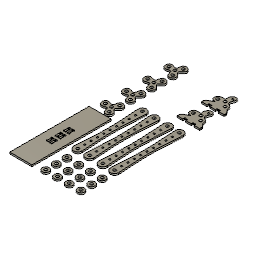
yufeng-lamp-thing (Autodesk Fusion 360 design; units mm, degrees)
part number: 2025-10-18-16-30-31-717
Autodesk Fusion 360 part; units mm, degrees
box "BoxPrimitive1" add length 1219.2 width 2438.4 height 11.7856 placed x (0, -1, 0) y (1, 0, 0) z (0, 0, 1) at (-34.3572, 8.0961, 0) makes body 1
move_body "Move1" bodies 1 to x (1, 0, 0) y (0, 1, 0) z (0, 0, 1) at (-89.6703, 115.0941, 0)
move_body "Move2" bodies 1 to x (1, 0, 0) y (0, 1, 0) z (0, 0, 1) at (127.2488, 1.4769, 0)
move_body "Move3" bodies 1 to x (1, 0, 0) y (0, 1, 0) z (0, 0, 1) at (-10.4658, -136.055, 0)
sketch "ELBOW" plane through (0, 0, 0) normal (0, 0, 1) x (1, 0, 0)
  line L0 (222.5472, -135.4361) -> (185.0472, -70.4842) construction
  line L1 (185.0472, -70.4842) -> (147.5472, -135.4361) construction
  line L2 (147.5472, -135.4361) -> (222.5472, -135.4361) construction
  circle A0 centre (185.0472, -70.4842) radius 25 construction
  circle A1 centre (147.5472, -135.4361) radius 25 construction
  circle A2 centre (222.5472, -135.4361) radius 25 construction
  line L3 (147.5472, -135.4361) -> (122.5472, -135.4361) construction
  line L4 (147.5472, -135.4361) -> (135.0472, -157.0867) construction
  line L5 (185.0472, -70.4842) -> (172.5472, -48.8336) construction
  line L6 (185.0472, -70.4842) -> (197.5472, -48.8336) construction
  line L7 (222.5472, -135.4361) -> (235.0472, -157.0867) construction
  line L8 (222.5472, -135.4361) -> (247.5472, -135.4361) construction
  line L9 (160.0472, -70.4842) -> (210.0472, -70.4842) construction
  line L10 (135.0472, -113.7855) -> (160.0472, -157.0867) construction
  line L11 (235.0472, -113.7855) -> (210.0472, -157.0867) construction
  line L12 (222.5472, -135.4361) -> (166.2972, -102.9601) construction
  line L13 (147.5472, -135.4361) -> (203.7972, -102.9601) construction
  line L14 (185.0472, -70.4842) -> (185.0472, -135.4361) construction
  spline S0 degree 5 poles (135.0472, -113.7855) (136.2523, -113.2432) (138.7814, -112.2557) (142.8843, -111.0513) (148.7127, -109.8794) (155.7527, -108.6478) (161.6818, -107.0834) (165.7867, -104.6636) (167.6575, -101.0152) (167.4018, -96.0557) (165.6038, -89.9888) (163.1024, -83.1934) (160.8198, -76.1444) (159.5754, -69.3217) (159.8917, -63.1196) (161.8468, -57.7723) (165.2277, -53.3996) (169.6524, -50.0384) (174.6931, -47.6782) (180.0245, -46.2985) (185.4687, -45.8896) (190.9043, -46.448) (196.2048, -47.9783) (201.1762, -50.4916) (205.4677, -54.0091) (208.6506, -58.5364) (210.3608, -64.026) (210.421, -70.343) (208.9713, -77.23) (206.5972, -84.2719) (204.1437, -90.9845) (202.5341, -96.9015) (202.5772, -101.6663) (204.8014, -105.1107) (209.2243, -107.369) (215.3774, -108.8454) (222.513, -110.0767) (229.759, -111.6244) (236.2898, -113.9581) (241.5029, -117.3331) (245.1562, -121.6999) (247.2527, -126.8142) (247.9512, -132.3267) (247.4748, -137.8722) (246.004, -143.1792) (243.6359, -148.0984) (240.4346, -152.5265) (236.459, -156.3518) (231.7968, -159.4005) (226.6048, -161.3583) (221.0926, -161.8511) (215.4834, -160.5874) (209.9826, -157.481) (204.7431, -152.782) (199.8317, -147.2051) (195.2451, -141.724) (190.9257, -137.3715) (186.7777, -135.0265) (182.6827, -135.2305) (178.5155, -137.9316) (174.1603, -142.5222) (169.5261, -148.0862) (164.5628, -153.5876) (159.2764, -158.0765) (153.7471, -160.9037) (148.1386, -161.8842) (142.6612, -161.1426) (137.5381, -158.9913) (132.9737, -155.806) (129.1131, -151.8787) (126.0369, -147.3683) (123.8027, -142.3818) (122.4778, -137.0263) (122.1686, -131.4643) (123.0691, -125.989) (125.3984, -120.9688) (128.5177, -117.5882) (131.5508, -115.5095) (133.8421, -114.3278) (135.0472, -113.7855) knots 0 0 0 0 0 0 0.01333333 0.02666667 0.04 0.05333333 0.06666667 0.08 0.09333333 0.10666667 0.12 0.13333333 0.14666667 0.16 0.17333333 0.18666667 0.2 0.21333333 0.22666667 0.24 0.25333333 0.26666667 0.28 0.29333333 0.30666667 0.32 0.33333333 0.34666667 0.36 0.37333333 0.38666667 0.4 0.41333333 0.42666667 0.44 0.45333333 0.46666667 0.48 0.49333333 0.50666667 0.52 0.53333333 0.54666667 0.56 0.57333333 0.58666667 0.6 0.61333333 0.62666667 0.64 0.65333333 0.66666667 0.68 0.69333333 0.70666667 0.72 0.73333333 0.74666667 0.76 0.77333333 0.78666667 0.8 0.81333333 0.82666667 0.84 0.85333333 0.86666667 0.88 0.89333333 0.90666667 0.92 0.93333333 0.94666667 0.96 0.97333333 0.98666667 1 1 1 1 1 1
  circle A3 centre (185.0472, -113.7855) radius 10.3
  circle A4 centre (185.0472, -70.4842) radius 10.3
  circle A5 centre (147.5472, -135.4361) radius 10.3
  circle A6 centre (222.5472, -135.4361) radius 10.3
  point P0 (185.0472, -113.7855)
  dimension "d13" = 75
  dimension "d14" = 50
  dimension "d15" = 50
  dimension "d16" = 50
  dimension "d19" = 20.6
  dimension "d20" = 20.6
  dimension "d21" = 20.6
  dimension "d22" = 20.6
  constraint coincident L0.end L1.start
  constraint coincident L1.end L2.start
  constraint coincident L0.start L2.end
  constraint coincident A1 L3.end
  constraint parallel L2 L3
  constraint coincident A1 L4.end
  constraint parallel L1 L4
  constraint coincident A0 L5.end
  constraint coincident A0 L6.end
  constraint coincident A2 L7.end
  constraint coincident A2 L8.end
  constraint parallel L2 L8
  constraint parallel L0 L7
  constraint parallel L0 L5
  constraint parallel L1 L6
  constraint coincident A0 L9.start
  constraint coincident A0 L9.end
  constraint coincident L0.end L9
  constraint coincident A1 L10.start
  constraint coincident A1 L10.end
  constraint coincident L1.end L10
  constraint parallel L0 L10
  constraint coincident A2 L11.start
  constraint coincident A2 L11.end
  constraint coincident L0.start L11
  constraint parallel L1 L11
  constraint midpoint L1 L12.end
  constraint midpoint L0 L13.end
  constraint midpoint L2 L14.end
  constraint coincident P0 A3.centre
  constraint concentric A0 A4
  constraint concentric A1 A5
  constraint concentric A2 A6
  measures "d13" distance of L0.start L0.end
  measures "d14" diameter of A0
  measures "d15" diameter of A1
  measures "d16" diameter of A2
  measures "d19" diameter of A3
  measures "d20" diameter of A4
  measures "d21" diameter of A5
  measures "d22" diameter of A6
sketch "SHOULDER" plane through (0, 0, 0) normal (0, 0, 1) x (1, 0, 0)
  line L0 (198.7656, -146.7949) -> (216.7517, -129.431) construction
  circle A0 centre (198.7656, -146.7949) radius 25 construction
  line L1 (198.7656, -146.7949) -> (180.8533, -209.228) construction
  line L2 (150.852, -223.1446) -> (138.763, -174.6281) construction
  circle A1 centre (216.8991, -219.5697) radius 25 construction
  line L3 (198.7656, -146.7949) -> (192.7211, -122.5366) construction
  line L4 (216.8991, -219.5697) -> (222.9436, -243.828) construction
  circle A2 centre (144.8075, -198.8864) radius 25 construction
  circle A3 centre (198.7656, -146.7949) radius 6
  line L5 (216.8991, -219.5697) -> (198.7656, -146.7949) construction
  circle A4 centre (186.8241, -188.417) radius 10.3
  line L6 (144.8075, -198.8864) -> (216.8991, -219.5697) construction
  line L7 (198.7656, -146.7949) -> (144.8075, -198.8864) construction
  circle A5 centre (144.8075, -198.8864) radius 10.3
  line L8 (144.8075, -198.8864) -> (207.8324, -183.1823) construction
  line L9 (198.9131, -236.9335) -> (234.8852, -202.2059) construction
  line L10 (216.8991, -219.5697) -> (240.9297, -226.4642) construction
  circle A6 centre (216.8991, -219.5697) radius 10.3
  line L11 (144.8075, -198.8864) -> (162.7936, -181.5225) construction
  line L12 (144.8075, -198.8864) -> (168.8381, -205.7808) construction
  line L13 (174.7351, -139.9004) -> (222.7962, -153.6893) construction
  line L14 (216.8991, -219.5697) -> (171.7866, -172.8406) construction
  line L15 (162.1875, -260.9179) -> (202.1875, -260.9179)
  line L16 (202.1875, -260.9179) -> (202.1875, -272.7035)
  line L17 (202.1875, -272.7035) -> (162.1875, -272.7035)
  line L18 (162.1875, -272.7035) -> (162.1875, -260.9179)
  line L19 (222.1875, -260.9179) -> (262.1875, -260.9179)
  line L20 (262.1875, -260.9179) -> (262.1875, -272.7035)
  line L21 (262.1875, -272.7035) -> (222.1875, -272.7035)
  line L22 (222.1875, -272.7035) -> (222.1875, -260.9179)
  line L23 (77.4298, -260.9179) -> (487.108, -260.9179) construction
  line L24 (202.1875, -272.7035) -> (222.1875, -272.7035) construction
  line L25 (142.1875, -260.9179) -> (102.1875, -260.9179)
  line L26 (102.1875, -260.9179) -> (102.1875, -272.7035)
  line L27 (102.1875, -272.7035) -> (142.1875, -272.7035)
  line L28 (142.1875, -272.7035) -> (142.1875, -260.9179)
  line L29 (142.1875, -272.7035) -> (162.1875, -272.7035) construction
  line L30 (144.8075, -198.8864) -> (126.8215, -216.2502) construction
  line L31 (198.7656, -146.7949) -> (205.6601, -122.7643) construction
  spline S0 degree 5 poles (102.1875, -260.9179) (102.2849, -259.2468) (103.2651, -255.7928) (106.9682, -250.3564) (115.5097, -242.9876) (128.9516, -234.6615) (141.5518, -228.1812) (150.0882, -224.1341) (152.4131, -222.5179) (148.2876, -222.4462) (139.793, -222.0811) (130.0596, -219.5224) (122.347, -213.4483) (118.7944, -204.075) (120.0937, -193.0921) (125.9149, -182.7571) (135.1188, -175.1879) (146.0593, -171.659) (156.8339, -171.6806) (165.6346, -173.346) (171.1696, -174.2996) (172.9964, -172.4342) (172.0506, -166.867) (170.5131, -158.1824) (170.8064, -147.7907) (174.8616, -137.5231) (183.1654, -129.1031) (194.2262, -123.759) (205.562, -122.2519) (214.5043, -124.841) (218.9994, -131.2846) (218.5854, -140.7942) (214.7048, -152.1106) (209.7356, -163.8008) (206.3147, -174.5033) (206.531, -183.1995) (211.2058, -189.4625) (219.0451, -193.7494) (227.5774, -197.0651) (234.2957, -200.5604) (237.5908, -205.1913) (238.1056, -211.2613) (238.1252, -218.4991) (240.0868, -226.3738) (245.375, -234.333) (252.9862, -242.0751) (260.4195, -249.4644) (264.586, -256.4485) (262.6599, -262.9794) (253.0747, -268.9202) (236.0664, -273.9998) (213.1247, -277.8807) (186.6627, -280.2049) (159.6018, -280.6485) (134.9944, -278.9721) (115.6308, -275.0743) (106.0484, -270.2493) (102.6812, -265.8194) (102.0902, -262.589) (102.1875, -260.9179) knots 0 0 0 0 0 0 0.018182 0.036364 0.054545 0.072727 0.090909 0.109091 0.127273 0.145455 0.163636 0.181818 0.2 0.218182 0.236364 0.254545 0.272727 0.290909 0.309091 0.327273 0.345455 0.363636 0.381818 0.4 0.418182 0.436364 0.454545 0.472727 0.490909 0.509091 0.527273 0.545455 0.563636 0.581818 0.6 0.618182 0.636364 0.654545 0.672727 0.690909 0.709091 0.727273 0.745455 0.763636 0.781818 0.8 0.818182 0.836364 0.854545 0.872727 0.890909 0.909091 0.927273 0.945455 0.963636 0.981818 1 1 1 1 1 1
  line L32 (142.1875, -260.9179) -> (162.1875, -260.9179)
  line L33 (202.1875, -260.9179) -> (222.1875, -260.9179)
  circle A7 centre (145.3625, -260.9175) radius 3.175
  circle A8 centre (159.0126, -260.9319) radius 3.175
  circle A9 centre (205.3625, -260.9179) radius 3.175
  circle A10 centre (219.0126, -260.9368) radius 3.175
  point P0 (186.8241, -188.417)
  dimension "d25" = 75
  dimension "d26" = 50
  dimension "d27" = 50
  dimension "d28" = 50
  dimension "d29" = 20.6
  dimension "d30" = 20.6
  dimension "d31" = 20.6
  dimension "d32" = 12
  dimension "d33" = 11.7856
  dimension "d34" = 11.7856
  dimension "d37" = 40
  dimension "d38" = 40
  dimension "d39" = 20
  dimension "d40" = 40
  dimension "d41" = 11.7856
  dimension "d42" = 20
  dimension "d269" = 6.35
  dimension "d270" = 6.35
  dimension "d271" = 6.35
  dimension "d272" = 6.35
  constraint coincident A2.centre L6.start
  constraint coincident A1.centre L4.start
  constraint coincident L0.start A0.centre
  constraint coincident L4.end A1
  constraint parallel L4 L5
  constraint coincident L10.end A1
  constraint parallel L6 L10
  constraint coincident L11.end A2
  constraint coincident L12.end A2
  constraint coincident L0.end A0
  constraint coincident L3.end A0
  constraint parallel L3 L5
  constraint parallel L0 L7
  constraint parallel L7 L11
  constraint parallel L6 L12
  constraint coincident L2.start A2
  constraint coincident L2.end A2
  constraint coincident A2.centre L2
  constraint coincident L9.start A1
  constraint coincident L9.end A1
  constraint coincident A1.centre L9
  constraint parallel L7 L9
  constraint coincident L13.start A0
  constraint coincident L13.end A0
  constraint coincident L0.start L13
  constraint parallel L6 L13
  constraint midpoint L1.end L6
  constraint midpoint L14.end L7
  constraint midpoint L8.end L5
  constraint coincident P0 A4.centre
  constraint concentric A2 A5
  constraint concentric A1 A6
  constraint concentric A0 A3
  constraint coincident L19 L23.end
  constraint coincident L15.start L23
  constraint coincident L23 L25.start
  constraint parallel L2 L5
  constraint coincident A2 L30.end
  constraint parallel L7 L30
  constraint coincident A0 L31.end
  constraint perpendicular L6 L31
  constraint coincident L25.start A7
  constraint coincident L15.start A8
  constraint coincident L15.end A9
  constraint coincident L19.start A10
  constraint coincident L19.end L23
  measures "d25" distance of L0.start A2.centre
  measures "d26" diameter of A2
  measures "d27" diameter of A1
  measures "d28" diameter of A0
  measures "d29" diameter of A4
  measures "d30" diameter of A5
  measures "d31" diameter of A6
  measures "d32" diameter of A3
  measures "d33" distance of L15.start L17.end
  measures "d34" distance of L19.start L21.end
  measures "d37" distance of L16.end L17.end
  measures "d38" distance of L20.end L21.end
  measures "d39" distance of L16.end L21.end
  measures "d40" distance of L25.start L25.end
  measures "d41" distance of L25.start L27.end
  measures "d42" distance of L17.end L27.end
  measures "d269" diameter of A7
  measures "d270" diameter of A8
  measures "d271" diameter of A9
  measures "d272" diameter of A10
sketch "BASE" plane through (0, 0, 0) normal (0, 0, 1) x (1, 0, 0)
  line L0 (-314.2507, -344.3749) -> (-355.2507, -344.3749)
  line L1 (-355.2507, -344.3749) -> (-355.2507, -331.5893)
  line L2 (-355.2507, -331.5893) -> (-314.2507, -331.5893)
  line L3 (-314.2507, -331.5893) -> (-314.2507, -344.3749)
  line L4 (-355.2507, -344.3749) -> (-375.2507, -344.3749) construction
  line L5 (-375.2507, -344.3749) -> (-375.2507, -331.5893)
  line L6 (-375.2507, -331.5893) -> (-355.2507, -331.5893) construction
  line L7 (-355.2507, -331.5893) -> (-355.2507, -344.3749)
  line L8 (-375.2507, -344.3749) -> (-416.2507, -344.3749)
  line L9 (-416.2507, -344.3749) -> (-416.2507, -331.5893)
  line L10 (-416.2507, -331.5893) -> (-375.2507, -331.5893)
  line L11 (-375.2507, -331.5893) -> (-375.2507, -344.3749)
  line L12 (-416.2507, -344.3749) -> (-436.2507, -344.3749) construction
  line L13 (-436.2507, -344.3749) -> (-436.2507, -331.5893)
  line L14 (-436.2507, -331.5893) -> (-416.2507, -331.5893) construction
  line L15 (-416.2507, -331.5893) -> (-416.2507, -344.3749)
  line L16 (-436.2507, -344.3749) -> (-477.2507, -344.3749)
  line L17 (-477.2507, -344.3749) -> (-477.2507, -331.5893)
  line L18 (-477.2507, -331.5893) -> (-436.2507, -331.5893)
  line L19 (-436.2507, -331.5893) -> (-436.2507, -344.3749)
  line L20 (-375.2507, -319.8037) -> (-416.2507, -319.8037)
  line L21 (-416.2507, -319.8037) -> (-436.2507, -319.8037) construction
  line L22 (-416.2507, -307.0181) -> (-375.2507, -307.0181)
  line L23 (-436.2507, -307.0181) -> (-436.2507, -319.8037)
  line L24 (-477.2507, -319.8037) -> (-477.2507, -307.0181)
  line L25 (-436.2507, -319.8037) -> (-436.2507, -307.0181)
  line L26 (-416.2507, -307.0181) -> (-416.2507, -319.8037)
  line L27 (-416.2507, -319.8037) -> (-416.2507, -307.0181)
  line L28 (-355.2507, -307.0181) -> (-314.2507, -307.0181)
  line L29 (-436.2507, -307.0181) -> (-416.2507, -307.0181) construction
  line L30 (-477.2507, -307.0181) -> (-436.2507, -307.0181)
  line L31 (-355.2507, -319.8037) -> (-375.2507, -319.8037) construction
  line L32 (-375.2507, -307.0181) -> (-375.2507, -319.8037)
  line L33 (-355.2507, -319.8037) -> (-355.2507, -307.0181)
  line L34 (-314.2507, -319.8037) -> (-355.2507, -319.8037)
  line L35 (-375.2507, -319.8037) -> (-375.2507, -307.0181)
  line L36 (-375.2507, -307.0181) -> (-355.2507, -307.0181) construction
  line L37 (-355.2507, -307.0181) -> (-355.2507, -319.8037)
  line L38 (-314.2507, -307.0181) -> (-314.2507, -319.8037)
  line L39 (-436.2507, -319.8037) -> (-477.2507, -319.8037)
  line L40 (-314.2507, -331.5893) -> (-314.2507, -319.8037)
  line L41 (-118.4603, -319.9195) -> (-329.7148, -319.9195) construction
  line L42 (-314.2507, -344.3749) -> (-114.2507, -344.3749) construction
  line L43 (-114.2507, -344.3749) -> (-114.2507, -404.3749)
  line L44 (-114.2507, -404.3749) -> (-314.2507, -404.3749)
  line L45 (-314.2507, -404.3749) -> (-314.2507, -344.3749) construction
  line L46 (-477.2507, -307.0181) -> (-677.2507, -307.0181) construction
  line L47 (-677.2507, -307.0181) -> (-677.2507, -247.0181)
  line L48 (-677.2507, -247.0181) -> (-477.2507, -247.0181)
  line L49 (-477.2507, -247.0181) -> (-477.2507, -307.0181) construction
  line L50 (-114.2507, -404.3749) -> (-677.2507, -404.3749)
  line L51 (-677.2507, -404.3749) -> (-677.2507, -247.0181)
  line L52 (-677.2507, -247.0181) -> (-114.2507, -247.0181)
  line L53 (-114.2507, -247.0181) -> (-114.2507, -404.3749)
  arc A0 (-477.2507, -344.3749) -> (-470.9225, -344.3749) centre (-474.0866, -344.1118) ccw
  circle A1 centre (-352.0757, -319.8037) radius 3.175
  circle A2 centre (-317.4257, -319.8037) radius 3.175
  arc A3 (-348.9022, -307.0181) -> (-355.2507, -307.0181) centre (-352.0765, -306.948) ccw
  arc A4 (-314.2507, -307.0181) -> (-320.5997, -307.0181) centre (-317.4252, -307.075) ccw
  arc A5 (-314.2507, -331.5893) -> (-320.5982, -331.5893) centre (-317.4244, -331.6788) ccw
  arc A6 (-320.5972, -344.3749) -> (-314.2507, -344.3749) centre (-317.4239, -344.4806) ccw
  arc A7 (-355.2507, -344.3749) -> (-348.9057, -344.3749) centre (-352.0782, -344.2491) ccw
  arc A8 (-348.9044, -331.5893) -> (-355.2507, -331.5893) centre (-352.0775, -331.4804) ccw
  arc A9 (-375.2507, -331.5893) -> (-381.5955, -331.5893) centre (-378.4231, -331.7174) ccw
  arc A10 (-381.5974, -319.8037) -> (-375.2507, -319.8037) centre (-378.424, -319.9063) ccw
  arc A11 (-375.2507, -307.0181) -> (-381.5987, -307.0181) centre (-378.4247, -307.0971) ccw
  arc A12 (-409.9038, -307.0181) -> (-416.2507, -307.0181) centre (-413.0773, -306.9179) ccw
  arc A13 (-416.2507, -319.8037) -> (-409.9056, -319.8037) centre (-413.0782, -319.6784) ccw
  arc A14 (-409.9083, -331.5893) -> (-416.2507, -331.5893) centre (-413.0795, -331.4343) ccw
  arc A15 (-381.594, -344.3749) -> (-375.2507, -344.3749) centre (-378.4223, -344.5208) ccw
  arc A16 (-416.2507, -344.3749) -> (-409.9104, -344.3749) centre (-413.0805, -344.1994) ccw
  arc A17 (-442.5868, -344.3749) -> (-436.2507, -344.3749) centre (-439.4187, -344.5846) ccw
  arc A18 (-436.2507, -331.5893) -> (-442.5899, -331.5893) centre (-439.4203, -331.7743) ccw
  arc A19 (-442.5935, -319.8037) -> (-436.2507, -319.8037) centre (-439.4221, -319.9543) ccw
  arc A20 (-436.2507, -307.0181) -> (-442.5961, -307.0181) centre (-439.4234, -307.1383) ccw
  arc A21 (-470.9075, -307.0181) -> (-477.2507, -307.0181) centre (-474.0791, -306.8706) ccw
  arc A22 (-477.2507, -319.8037) -> (-470.9121, -319.8037) centre (-474.0814, -319.6133) ccw
  arc A23 (-470.9167, -331.5893) -> (-477.2507, -331.5893) centre (-474.0837, -331.3638) ccw
  dimension "d45" = 41
  dimension "d46" = 12.7856
  dimension "d47" = 20
  dimension "d48" = 12.7856
  dimension "d49" = 41
  dimension "d50" = 12.7856
  dimension "d51" = 20
  dimension "d52" = 12.7856
  dimension "d53" = 41
  dimension "d54" = 12.7856
  dimension "d55" = 41
  dimension "d56" = 12.7856
  dimension "d57" = 20
  dimension "d58" = 12.7856
  dimension "d59" = 41
  dimension "d60" = 12.7856
  dimension "d61" = 20
  dimension "d62" = 12.7856
  dimension "d63" = 41
  dimension "d64" = 12.7856
  dimension "d65" = 11.7856
  dimension "d66" = 60
  dimension "d67" = 200
  dimension "d70" = 200
  dimension "d71" = 60
  dimension "d284" = 6.35
  dimension "d285" = 6.35
  dimension "d286" = 6.35
  dimension "d287" = 6.35
  dimension "d288" = 6.35
  dimension "d289" = 6.35
  dimension "d290" = 6.35
  dimension "d291" = 6.35
  dimension "d292" = 6.35
  dimension "d293" = 6.35
  dimension "d294" = 6.35
  dimension "d295" = 6.35
  dimension "d296" = 6.35
  dimension "d297" = 6.35
  dimension "d298" = 6.35
  dimension "d299" = 6.35
  dimension "d300" = 6.35
  dimension "d301" = 6.35
  dimension "d302" = 6.35
  dimension "d303" = 6.35
  dimension "d304" = 6.35
  dimension "d305" = 6.35
  dimension "d306" = 6.35
  dimension "d307" = 6.35
  constraint horizontal L0
  constraint vertical L1
  constraint horizontal L2
  constraint vertical L3
  constraint horizontal L4
  constraint vertical L5
  constraint horizontal L6
  constraint vertical L7
  constraint horizontal L8
  constraint vertical L9
  constraint horizontal L10
  constraint vertical L11
  constraint horizontal L12
  constraint vertical L13
  constraint horizontal L14
  constraint vertical L15
  constraint horizontal L16
  constraint vertical L17
  constraint horizontal L18
  constraint vertical L19
  constraint horizontal L34
  constraint vertical L33
  constraint horizontal L28
  constraint vertical L38
  constraint horizontal L31
  constraint vertical L35
  constraint horizontal L36
  constraint vertical L37
  constraint horizontal L20
  constraint vertical L27
  constraint horizontal L22
  constraint vertical L32
  constraint horizontal L21
  constraint vertical L25
  constraint horizontal L29
  constraint vertical L26
  constraint horizontal L39
  constraint vertical L24
  constraint horizontal L30
  constraint vertical L23
  constraint perpendicular L34 L40
  constraint horizontal L42
  constraint vertical L43
  constraint horizontal L44
  constraint vertical L45
  constraint horizontal L46
  constraint vertical L47
  constraint horizontal L48
  constraint vertical L49
  constraint horizontal L50
  constraint vertical L51
  constraint horizontal L52
  constraint vertical L53
  constraint coincident L16 A0.end
  constraint coincident L23.start A20
  constraint coincident L22.start A12
  constraint coincident L9.end A14
  constraint coincident L5.end A9
  constraint coincident L13.end A18
  constraint coincident L28.start A3
  constraint coincident L31.start A1
  constraint coincident L1.end A8
  constraint coincident L34.start A2
  constraint coincident L28 A3.start
  constraint coincident L28 A4.end
  constraint coincident L2 A5.end
  constraint coincident L0 A6.start
  constraint coincident L0 A7.end
  constraint coincident L2 A8.start
  constraint coincident L10 A9.end
  constraint coincident L20 A10.start
  constraint coincident L22 A11.end
  constraint coincident L22 A12.start
  constraint coincident L20 A13.end
  constraint coincident L10 A14.start
  constraint coincident L8 A15.start
  constraint coincident L8 A16.end
  constraint coincident L16 A17.start
  constraint coincident L18 A18.end
  constraint coincident L39 A19.start
  constraint coincident L30 A20.end
  constraint coincident L30 A21.start
  constraint coincident L39 A22.end
  constraint coincident L18 A23.start
  measures "d45" distance of L0.start L0.end
  measures "d46" distance of L0.start L2.end
  measures "d47" distance of L0.end L4.end
  measures "d48" distance of L0.end L1.end
  measures "d49" distance of L4.end L8.end
  measures "d50" distance of L4.end L5.end
  measures "d51" distance of L8.end L12.end
  measures "d52" distance of L8.end L9.end
  measures "d53" distance of L12.end L16.end
  measures "d54" distance of L12.end L13.end
  measures "d55" distance of L31.start L34.start
  measures "d56" distance of L28.end L34.start
  measures "d57" distance of L31.start L20.start
  measures "d58" distance of L31.start L28.start
  measures "d59" distance of L20.end L20.start
  measures "d60" distance of L22.end L20.start
  measures "d61" distance of L20.end L21.end
  measures "d62" distance of L20.end L22.start
  measures "d63" distance of L24.start L21.end
  measures "d64" distance of L23.start L21.end
  measures "d65" distance of L2.end L34.start
  measures "d66" distance of L0.start L44.end
  measures "d67" distance of L43.end L44.end
  measures "d70" distance of L24.end L46.end
  measures "d71" distance of L24.end L48.end
  measures "d284" diameter of A0
  measures "d285" diameter of A23
  measures "d286" diameter of A22
  measures "d287" diameter of A21
  measures "d288" diameter of A20
  measures "d289" diameter of A19
  measures "d290" diameter of A12
  measures "d291" diameter of A13
  measures "d292" diameter of A11
  measures "d293" diameter of A10
  measures "d294" diameter of A14
  measures "d295" diameter of A16
  measures "d296" diameter of A9
  measures "d297" diameter of A15
  measures "d298" diameter of A18
  measures "d299" diameter of A17
  measures "d300" diameter of A3
  measures "d301" diameter of A1
  measures "d302" diameter of A8
  measures "d303" diameter of A7
  measures "d304" diameter of A4
  measures "d305" diameter of A5
  measures "d306" diameter of A2
  measures "d307" diameter of A6
ref_plane "WorkPlane1" through (302.5055, -90.1825, 0) normal (0, 0, 1) x (1, 0, 0)
ref_plane "WorkPlane2" through (302.5055, -102.5225, 0) normal (0, 0, 1) x (1, 0, 0)
ref_plane "WorkPlane3" through (342.5055, -102.5225, 0) normal (0, 0, 1) x (1, 0, 0)
ref_plane "WorkPlane4" through (342.5055, -90.1825, 0) normal (0, 0, 1) x (1, 0, 0)
ref_plane "WorkPlane5" through (422.5055, -77.8425, 0) normal (0, 0, 1) x (1, 0, 0)
ref_plane "WorkPlane6" through (462.5055, -77.8425, 0) normal (0, 0, 1) x (1, 0, 0)
ref_plane "WorkPlane7" through (462.5055, -65.5025, 0) normal (0, 0, 1) x (1, 0, 0)
ref_plane "WorkPlane8" through (422.5055, -65.5025, 0) normal (0, 0, 1) x (1, 0, 0)
ref_plane "WorkPlane9" through (422.5055, -90.1825, 0) normal (0, 0, 1) x (1, 0, 0)
ref_plane "WorkPlane10" through (422.5055, -102.5225, 0) normal (0, 0, 1) x (1, 0, 0)
ref_plane "WorkPlane11" through (462.5055, -102.5225, 0) normal (0, 0, 1) x (1, 0, 0)
ref_plane "WorkPlane12" through (462.5055, -90.1825, 0) normal (0, 0, 1) x (1, 0, 0)
ref_plane "WorkPlane13" through (362.5055, -90.1825, 0) normal (0, 0, 1) x (1, 0, 0)
ref_plane "WorkPlane14" through (362.5055, -102.5225, 0) normal (0, 0, 1) x (1, 0, 0)
ref_plane "WorkPlane15" through (402.5055, -102.5225, 0) normal (0, 0, 1) x (1, 0, 0)
ref_plane "WorkPlane16" through (402.5055, -90.1825, 0) normal (0, 0, 1) x (1, 0, 0)
ref_plane "WorkPlane17" through (402.5055, -77.8425, 0) normal (0, 0, 1) x (1, 0, 0)
ref_plane "WorkPlane18" through (402.5055, -65.5025, 0) normal (0, 0, 1) x (1, 0, 0)
ref_plane "WorkPlane19" through (362.5055, -65.5025, 0) normal (0, 0, 1) x (1, 0, 0)
ref_plane "WorkPlane20" through (362.5055, -77.8425, 0) normal (0, 0, 1) x (1, 0, 0)
ref_plane "WorkPlane21" through (342.5055, -65.5025, 0) normal (0, 0, 1) x (1, 0, 0)
ref_plane "WorkPlane22" through (302.5055, -65.5025, 0) normal (0, 0, 1) x (1, 0, 0)
ref_plane "WorkPlane23" through (302.5055, -77.8425, 0) normal (0, 0, 1) x (1, 0, 0)
ref_plane "WorkPlane24" through (342.5055, -77.8425, 0) normal (0, 0, 1) x (1, 0, 0)
ref_plane "WorkPlane25" through (583.562, -149.703, 0) normal (0, 0, 1) x (1, 0, 0)
extrude "Extrude5" add sketch "SHOULDER" along normal blind 11.7856 separate body contours L15 L19 L25 S0 L32 L33 A7 A8 A9 A10 | L15 L16 L17 L18 A8 | L25 L26 L27 L28 S0 | L19 L21 L22 S0 A10 | L20 L21 S0 | L26 L27 S0 makes body 2
move_body "Move8" bodies 2 to x (1, 0, 0) y (0, 1, 0) z (0, 0, 1) at (3.7993, 52.1795, 0)
extrude "Extrude6" add sketch "BASE" along normal blind 11.7856 separate body makes body 3
sketch "SPACER" plane through (0, 0, 0) normal (0, 0, 1) x (1, 0, 0)
  circle A0 centre (55.9986, -45.1226) radius 25
  circle A1 centre (55.9986, -45.1226) radius 10.3
  dimension "d310" = 50
  dimension "d311" = 20.6
  constraint concentric A0 A1
  measures "d310" diameter of A0
  measures "d311" diameter of A1
extrude "Extrude7" add sketch "SPACER" along normal blind 11.7856 separate body makes body 4
extrude "Extrude8" add sketch "ELBOW" along normal blind 11.7856 separate body makes body 5
sketch "ARM" plane through (0, 0, 0) normal (0, 0, 1) x (1, 0, 0)
  line L0 (63.2655, -241.1973) -> (520.4655, -241.1973) construction
  line L1 (520.4655, -241.1973) -> (520.4655, -301.1973) construction
  line L2 (520.4655, -301.1973) -> (63.2655, -301.1973) construction
  line L3 (63.2655, -301.1973) -> (63.2655, -241.1973) construction
  circle A0 centre (63.2655, -271.1973) radius 10.3
  circle A1 centre (520.4655, -271.1973) radius 10.3
  line L4 (291.8655, -241.1973) -> (291.8655, -301.1973) construction
  circle A2 centre (291.8655, -271.1973) radius 6
  circle A3 centre (336.8655, -271.1973) radius 6
  circle A4 centre (381.8655, -271.1973) radius 6
  circle A5 centre (426.8655, -271.1973) radius 6
  circle A6 centre (471.8655, -271.1973) radius 6
  circle A7 centre (246.8655, -271.1973) radius 6
  circle A8 centre (201.8655, -271.1973) radius 6
  circle A9 centre (156.8655, -271.1973) radius 6
  circle A10 centre (111.8655, -271.1973) radius 6
  arc A11 (63.2655, -241.1973) -> (63.2655, -301.1973) centre (63.2655, -271.1973) ccw
  arc A12 (520.4655, -301.1973) -> (520.4655, -241.1973) centre (520.4655, -271.1973) ccw
  line L5 (291.8655, -241.1973) -> (291.8655, -256.1973) construction
  line L6 (291.8655, -301.1973) -> (291.8655, -286.1973) construction
  spline S0 degree 2 poles (63.2655, -241.1973) (291.8655, -256.1973) (520.4655, -241.1973) knots 0 0 0 45.775331 45.775331 45.775331 weights 1 3 1
  spline S1 degree 2 poles (63.2655, -301.1973) (291.8655, -286.1973) (520.4655, -301.1973) knots 0 0 0 45.775331 45.775331 45.775331 weights 1 3 1
  dimension "d317" = 457.2
  dimension "d318" = 20.6
  dimension "d319" = 20.6
  dimension "d320" = 12
  dimension "d328" = 180
  dimension "d329" = 0
  dimension "d333" = 0
  dimension "d334" = 60
  dimension "d335" = 15
  dimension "d336" = 15
  constraint horizontal L0
  constraint vertical L1
  constraint horizontal L2
  constraint vertical L3
  constraint midpoint L3 A0.centre
  constraint midpoint L1 A1.centre
  constraint coincident L0 L4.start
  constraint coincident L2 L4.end
  constraint perpendicular L2 L4
  constraint midpoint L0 L4.start
  constraint midpoint L4 A2.centre
  constraint tangent L2 A11
  constraint tangent L2 A12
  constraint perpendicular L0 L5
  constraint perpendicular L2 L6
  measures "d317" distance of L0.start L0.end
  measures "d318" diameter of A0
  measures "d319" diameter of A1
  measures "d320" diameter of A2
  measures "d334" distance of L0 L2
  measures "d335" distance of L4.start L5.end
  measures "d336" distance of L4.end L6.end
extrude "Extrude9" add sketch "ARM" along normal blind 11.7856 separate body makes body 6
move_body "Move9" bodies 2 to x (1, 0, 0) y (0, 1, 0) z (0, 0, 1) at (-27.2863, -253.1566, 0)
move_body "Move10" bodies 3 to x (1, 0, 0) y (0, 1, 0) z (0, 0, 1) at (-172.8135, -501.7655, 0)
move_body "Move11" bodies 4 to x (1, 0, 0) y (0, 1, 0) z (0, 0, 1) at (309.6954, -497.5434, 0)
move_body "Move12" bodies 5 to x (1, 0, 0) y (0, 1, 0) z (0, 0, 1) at (370.6191, -286.0029, 0)
move_body "Move13" bodies 6 to x (1, 0, 0) y (0, 1, 0) z (0, 0, 1) at (69.3853, 113.3857, 0)
pattern_linear "R-Pattern1" count 1 spacing 0 along (1, 0, 0) count 4 spacing 83.3333 along (0, -1, 0) of bodies 6 makes body 7 at (467.5357, -259.3931, 0) makes body 8 at (467.5357, -306.2301, 0) makes body 9 at (467.5357, -389.5634, 0)
move_body "Move14" bodies 9 8 7 6 to x (1, 0, 0) y (0, 1, 0) z (0, 0, 1) at (-54.1544, 64.3083, 0)
move_body "Move15" bodies 2 to x (1, 0, 0) y (0, 1, 0) z (0, 0, 1) at (533.0822, 264.0026, 0)
pattern_linear "R-Pattern2" count 1 spacing 0 along (1, 0, 0) count 2 spacing 150 along (0, -1, 0) of bodies 2 makes body 10
pattern_linear "R-Pattern3" count 4 spacing 150 along (1, 0, 0) of bodies 5 makes body 11 at (683.8039, -403.6119, 0) makes body 12 at (833.8039, -403.6119, 0) makes body 13 at (983.8039, -403.6119, 0)
move_body "Move16" bodies 5 12 13 11 to x (1, 0, 0) y (0, 1, 0) z (0, 0, 1) at (-441.6967, -52.4621, 0)
pattern_linear "R-Pattern4" count 4 spacing 83.3333 along (1, 0, 0) count 3 spacing 75 along (0, -1, 0) of bodies 4 makes body 14 at (472.0643, -532.9551, 7.8571) makes body 15 at (536.7019, -518.0458, 7.8571) makes body 16 at (620.0352, -518.0458, 7.8571) makes body 17 at (388.7309, -607.9551, 7.8571) makes body 18 at (472.0643, -607.9551, 7.8571) makes body 19 at (536.7019, -593.0458, 7.8571) makes body 20 at (620.0352, -593.0458, 7.8571) makes body 21 at (388.7309, -682.9551, 7.8571) makes body 22 at (472.0643, -682.9551, 7.8571) makes body 23 at (536.7019, -668.0458, 7.8571) makes body 24 at (620.0352, -668.0458, 7.8571)
move_body "Move17" bodies 4 15 20 21 16 19 22 14 17 18 23 24 to x (1, 0, 0) y (0, 1, 0) z (0, 0, 1) at (341.8496, 138.7706, 0)
move_body "Move18" bodies 3 to x (1, 0, 0) y (0, 1, 0) z (0, 0, 1) at (-5.077, -32.1542, 0)
move_body "Move19" bodies 22 4 10 23 19 24 5 11 14 7 8 12 9 2 20 17 15 13 6 18 1 16 3 21 to x (1, 0, 0) y (0, 1, 0) z (0, 0, 1) at (-2400, 0, 0)
move_body "Move20" bodies 2 6 3 15 5 7 9 8 4 20 21 12 10 16 19 22 13 14 17 18 11 23 24 to x (1, 0, 0) y (0, 1, 0) z (0, 0, 1) at (1400, 0, 0)
move_body "Move29" bodies 18 14 21 16 23 22 15 19 20 4 17 24 to x (1, 0, 0) y (0, 1, 0) z (0, 0, 1) at (12.6714, -617.962, 0)
move_body "Move30" bodies 5 12 11 13 to x (0, 1, 0) y (-1, 0, 0) z (0, 0, 1) at (-517.5443, -5.7443, 0)
move_body "Move31" bodies 2 10 to x (1, 0, 0) y (0, 1, 0) z (0, 0, 1) at (242.7329, 5.9706, 0)
move_body "Move32" bodies 6 7 to x (0, 1, 0) y (-1, 0, 0) z (0, 0, 1) at (-359.4303, 10.6712, 0)
move_body "Move33" bodies 8 9 to x (0, 1, 0) y (-1, 0, 0) z (0, 0, 1) at (-705.5818, 12.4458, 0)
move_body "Move34" bodies 13 5 12 11 to x (1, 0, 0) y (0, 1, 0) z (0, 0, 1) at (-1200, 0, 0)
move_body "Move35" bodies 9 7 8 6 to x (1, 0, 0) y (0, 1, 0) z (0, 0, 1) at (150, -20, 0)
move_body "Move36" bodies 3 to x (0, 1, 0) y (-1, 0, 0) z (0, 0, 1) at (-1008.0547, 654.0639, 0)
move_body "Move37" bodies 3 to x (1, 0, 0) y (0, 1, 0) z (0, 0, 1) at (160.209, -43.9034, 0)
move_body "Move38" bodies 3 to x (1, 0, 0) y (0, 1, 0) z (0, 0, 1) at (-166.6977, -561.002, 0)
move_body "Move40" bodies 3 to x (1, 0, 0) y (0, 1, 0) z (0, 0, 1) at (-281.9195, 613.8569, 0)
move_body "Move41" bodies 11 13 12 5 to x (1, 0, 0) y (0, 1, 0) z (0, 0, 1) at (834.1437, 337.0544, 0)
move_body "Move42" bodies 10 to x (1, 0, 0) y (0, 1, 0) z (0, 0, 1) at (-0.6198, -21.6931, 0)
hidden bodies 1
equation "stock_thickness = 0.464 in"
equation "stock_width = 1219.2 mm"
equation "stock_height = 2438.4 mm"
equation "d6 = stock_width"
equation "d7 = stock_height"
equation "d8 = stock_thickness"
equation "spinner_circle_diameter = 50 mm"
equation "spinner_circle_distance = spinner_circle_diameter * 1.5"
equation "d13 = spinner_circle_distance"
equation "d14 = spinner_circle_diameter"
equation "d15 = spinner_circle_diameter"
equation "d16 = spinner_circle_diameter"
equation "dowel_diameter_big = 19.6 mm"
equation "dowel_diameter_small = 11 mm"
equation "d19 = dowel_diameter_big + joint_tolerance"
equation "d20 = dowel_diameter_big + joint_tolerance"
equation "d21 = dowel_diameter_big + joint_tolerance"
equation "d22 = dowel_diameter_big + joint_tolerance"
equation "d25 = spinner_circle_distance"
equation "d26 = spinner_circle_diameter"
equation "d27 = spinner_circle_diameter"
equation "d28 = spinner_circle_diameter"
equation "d29 = dowel_diameter_big + joint_tolerance"
equation "d30 = dowel_diameter_big + joint_tolerance"
equation "d31 = dowel_diameter_big + joint_tolerance"
equation "d32 = dowel_diameter_small + joint_tolerance"
equation "d33 = stock_thickness"
equation "d34 = stock_thickness"
equation "shoulder_mount_gap = 20 mm"
equation "shoulder_mount_width = 40 mm"
equation "d37 = shoulder_mount_width"
equation "d38 = shoulder_mount_width"
equation "d39 = shoulder_mount_gap"
equation "d40 = shoulder_mount_width"
equation "d41 = stock_thickness"
equation "d42 = shoulder_mount_gap"
equation "d45 = shoulder_mount_width + joint_tolerance"
equation "d46 = stock_thickness + joint_tolerance"
equation "d47 = shoulder_mount_gap"
equation "d48 = stock_thickness + joint_tolerance"
equation "d49 = shoulder_mount_width + joint_tolerance"
equation "d50 = stock_thickness + joint_tolerance"
equation "d51 = shoulder_mount_gap"
equation "d52 = stock_thickness + joint_tolerance"
equation "d53 = shoulder_mount_width + joint_tolerance"
equation "d54 = stock_thickness + joint_tolerance"
equation "d55 = shoulder_mount_width + joint_tolerance"
equation "d56 = stock_thickness + joint_tolerance"
equation "d57 = shoulder_mount_gap"
equation "d58 = stock_thickness + joint_tolerance"
equation "d59 = shoulder_mount_width + joint_tolerance"
equation "d60 = stock_thickness + joint_tolerance"
equation "d61 = shoulder_mount_gap"
equation "d62 = stock_thickness + joint_tolerance"
equation "d63 = shoulder_mount_width + joint_tolerance"
equation "d64 = stock_thickness + joint_tolerance"
equation "d65 = stock_thickness"
equation "endmill_diameter = 0.25 in"
equation "dogbone_radial_offset = -2 mm"
equation "d269 = endmill_diameter"
equation "d270 = endmill_diameter"
equation "d271 = endmill_diameter"
equation "d272 = endmill_diameter"
equation "joint_tolerance = 1 mm"
equation "d276 = stock_thickness"
equation "d284 = endmill_diameter"
equation "d285 = endmill_diameter"
equation "d286 = endmill_diameter"
equation "d287 = endmill_diameter"
equation "d288 = endmill_diameter"
equation "d289 = endmill_diameter"
equation "d290 = endmill_diameter"
equation "d291 = endmill_diameter"
equation "d292 = endmill_diameter"
equation "d293 = endmill_diameter"
equation "d294 = endmill_diameter"
equation "d295 = endmill_diameter"
equation "d296 = endmill_diameter"
equation "d297 = endmill_diameter"
equation "d298 = endmill_diameter"
equation "d299 = endmill_diameter"
equation "d300 = endmill_diameter"
equation "d301 = endmill_diameter"
equation "d302 = endmill_diameter"
equation "d303 = endmill_diameter"
equation "d304 = endmill_diameter"
equation "d305 = endmill_diameter"
equation "d306 = endmill_diameter"
equation "d307 = endmill_diameter"
equation "d308 = stock_thickness"
equation "d310 = spinner_circle_diameter"
equation "d311 = dowel_diameter_big + joint_tolerance"
equation "d312 = stock_thickness"
equation "d314 = stock_thickness"
equation "arm_dowel_distance = 18 in"
equation "d317 = arm_dowel_distance"
equation "d318 = dowel_diameter_big + joint_tolerance"
equation "d319 = dowel_diameter_big + joint_tolerance"
equation "d320 = dowel_diameter_small + joint_tolerance"
equation "arm_hole_gap = 180 mm"
equation "d328 = arm_hole_gap"
equation "d332 = -arm_hole_gap"
equation "d340 = stock_thickness"
named bodies: "STOCK", "SHOULDER_B", "BASE_B", "SPACER_B", "ELBOW_B", "ARM_B", "ARM_B (1)", "ARM_B (2)", "ARM_B (3)", "SHOULDER_B (1)", "ELBOW_B (1)", "ELBOW_B (2)", "ELBOW_B (3)", "SPACER_B (1)", "SPACER_B (2)", "SPACER_B (3)", "SPACER_B (4)", "SPACER_B (5)", "SPACER_B (6)", "SPACER_B (7)", "SPACER_B (8)", "SPACER_B (9)", "SPACER_B (10)", "SPACER_B (11)"
